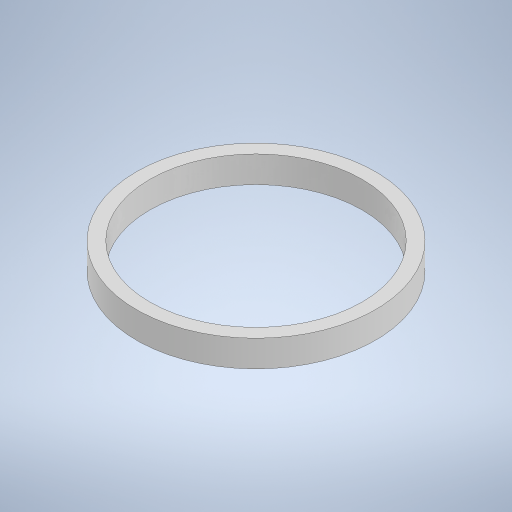
# Autodesk Inventor part: Adattatore
Saved by Autodesk Inventor 2024 (Build 280153000, 153)
## iProperties
Created: 2023-12-13
Part Number: Adattatore
Material: Generico
Document SubType Name: Modeling
Designer: Leonardo
Density: 1 g/cm^3
Appearance: Default
Author: Leonardo
Autodesk Inventor part; units mm, degrees
ref_plane "YZ Plane" through (0, 0, 0) normal (1, 0, 0) x (0, 1, 0)
ref_plane "XZ Plane" through (0, 0, 0) normal (0, 1, 0) x (-1, 0, 0)
ref_plane "XY Plane" through (0, 0, 0) normal (0, 0, 1) x (1, 0, 0)
sketch "Schizzo1" plane through (0, 0, 0) normal (0, 1, 0) x (-1, 0, 0)
  circle A0 centre (0, 0) radius 8
  circle A1 centre (0, 0) radius 9
  line L0 (-10, -10) -> (10, -10)
  line L1 (10, -10) -> (10, 10)
  line L2 (10, 10) -> (-10, 10)
  line L3 (-10, 10) -> (-10, -10)
  line L4 (-10, -10) -> (10, 10) construction
  line L5 (10, -10) -> (-10, 10) construction
  line L6 (9, 10) -> (-8, 10)
  line L7 (10, 10) -> (11, 10)
  line L8 (11, 9) -> (10, 9)
  line L9 (10, 9) -> (10, 10)
  line L10 (10, -10) -> (11, -10)
  line L11 (11, -9) -> (10, -9)
  line L12 (10, -9) -> (10, -10)
  line L13 (9, 10) -> (-9, 10)
  line L14 (-9, 10) -> (-9, 11)
  line L15 (-9, 11) -> (9, 11)
  line L16 (9, 11) -> (9, 10)
  line L17 (-10, 10) -> (-11, 10)
  line L18 (-11, 9) -> (-10, 9)
  line L19 (-10, 9) -> (-10, 10)
  line L20 (-10, -10) -> (-11, -10)
  line L21 (-11, -9) -> (-10, -9)
  line L22 (-10, -9) -> (-10, -10)
  line L23 (9, -10) -> (-9, -10)
  line L24 (-9, -10) -> (-9, -11)
  line L25 (-9, -11) -> (9, -11)
  line L26 (9, -11) -> (9, -10)
  line L27 (11, 10) -> (12, 10)
  line L28 (12, 10) -> (12, 8)
  line L29 (12, 8) -> (11, 8)
  line L30 (11, 9) -> (11, 8)
  line L31 (11, -10) -> (12, -10)
  line L32 (12, -10) -> (12, -8)
  line L33 (12, -8) -> (11, -8)
  line L34 (11, -8) -> (11, -9)
  line L35 (-11, -10) -> (-12, -10)
  line L36 (-12, -10) -> (-12, -8)
  line L37 (-12, -8) -> (-11, -8)
  line L38 (-11, -8) -> (-11, -9)
  line L39 (-11, 10) -> (-12, 10)
  line L40 (-12, 10) -> (-12, 8)
  line L41 (-12, 8) -> (-11, 8)
  line L42 (-11, 8) -> (-11, 9)
  dimension "d0" = 16
  dimension "d1" = 18
  dimension "d2" = 20
  dimension "d3" = 20
  dimension "d6" = 1
  dimension "d7" = 1
  dimension "d8" = 1
  dimension "d9" = 1
  dimension "d10" = 1
  dimension "d11" = 1
  dimension "d12" = 1
  dimension "d13" = 1
  dimension "d14" = 1
  dimension "d15" = 18
  dimension "d16" = 1
  dimension "d17" = 2
  dimension "d18" = 1
  dimension "d19" = 2
  dimension "d20" = 1
  dimension "d21" = 2
  dimension "d22" = 1
  dimension "d23" = 2
  constraints: 86 end point, 14 parallel, 12 horizontal, 7 perpendicular, 4 vertical, 2 centre point, 2 coincident, 2 midpoint, 2 point on line
  measures "d0" diameter of A0
  measures "d1" diameter of A1
  measures "d2" distance of L2.end L1.end
  measures "d3" distance of L1.end L0.end
  measures "d6" distance of L8.start L8.end
  measures "d7" distance of L7.end L8.start
  measures "d8" distance of L11.end L11.start
  measures "d9" distance of L11.start L10.end
  measures "d10" distance of L13.end L14.end
  measures "d11" distance of L18.end L18.start
  measures "d12" distance of L18.start L17.end
  measures "d13" distance of L21.start L21.end
  measures "d14" distance of L20.end L21.start
  measures "d15" distance of L25.end L24.end
  measures "d16" distance of L28.end L29.end
  measures "d17" distance of L27.end L28.end
  measures "d18" distance of L33.end L32.end
  measures "d19" distance of L32.end L31.end
  measures "d20" distance of L36.end L37.end
  measures "d21" distance of L35.end L36.end
  measures "d22" distance of L41.end L40.end
  measures "d23" distance of L40.end L39.end
extrude "Estrusione2" add sketch "Schizzo1" along normal blind 2 contours A1
